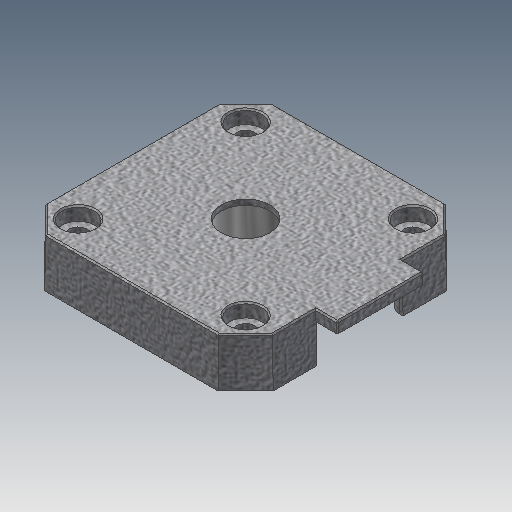
# Autodesk Inventor part: Nema 17 Base Cap
Saved by Autodesk Inventor 2020.2 (Build 242310000, 310)
## iProperties
Created: 2020-01-17
Part Number: Nema 17 Base Cap
Material: Aluminum 6061
Document SubType Name: Modeling
Designer: james
Density: 2.7 g/cm^3
Appearance: Aluminum Cast
Mass: 22.7 g
Surface Area: 71.1651 cm^2
Volume: 8.4074 cm^3
Author: james
Autodesk Inventor part; units mm, degrees
ref_plane "YZ Plane" through (0, 0, 0) normal (1, 0, 0) x (0, 1, 0)
ref_plane "XZ Plane" through (0, 0, 0) normal (0, 1, 0) x (-1, 0, 0)
ref_plane "XY Plane" through (0, 0, 0) normal (0, 0, 1) x (1, 0, 0)
sketch "Sketch11" plane through (0, 0, 0) normal (0, 1, 0) x (-1, 0, 0)
  line L0 (-16, 21) -> (16, 21)
  line L1 (21, 16) -> (21, -16)
  line L2 (16, -21) -> (-16, -21)
  line L3 (-21, -16) -> (-21, 16)
  line L4 (-21, 21) -> (21, -21) construction
  line L5 (21, 21) -> (-21, -21) construction
  line L6 (21, -16) -> (16, -21)
  line L7 (-16, -21) -> (-21, -16)
  line L8 (-21, 16) -> (-16, 21)
  line L9 (16, 21) -> (21, 16)
  point P0 (0, 0)
  dimension "d82" = 42
  dimension "d83" = 5
  dimension "d84" = 5
  dimension "d85" = 5
  dimension "d86" = 5
  dimension "d87" = 5
  dimension "d88" = 5
  dimension "d89" = 5
  dimension "d90" = 5
  constraints: 20 end point, 8 point on line, 2 midpoint, 2 parallel, 2 perpendicular, 1 horizontal
  measures "d82" distance between parallel lines of L0 L2
  measures "d83" distance of L1.end L4.end
  measures "d84" distance of L2.start L4.end
  measures "d85" distance of L2.end L5.end
  measures "d86" distance of L3.start L5.end
  measures "d87" distance of L3.end L4.start
  measures "d88" distance of L0.start L4.start
  measures "d89" distance of L0.end L5.start
  measures "d90" distance of L1.start L5.start
extrude "Extrusion7" add sketch "Sketch11" against normal blind 9 draft 1
sketch "Sketch13" plane through (0, -9, 0) normal (0, -1, 0) x (1, 0, 0)
  circle A0 centre (0, 0) radius 13
  line L0 (-8.0772, 19.5) -> (8.0772, 19.5)
  line L1 (8.0772, 19.5) -> (19.5, 8.0772)
  line L2 (19.5, 8.0772) -> (19.5, -8.0772)
  line L3 (19.5, -8.0772) -> (8.0772, -19.5)
  line L4 (8.0772, -19.5) -> (-8.0772, -19.5)
  line L5 (-8.0772, -19.5) -> (-19.5, -8.0772)
  line L6 (-19.5, -8.0772) -> (-19.5, 8.0772)
  line L7 (-19.5, 8.0772) -> (-8.0772, 19.5)
  dimension "d96" = 26
  dimension "d97" = 39
  constraints: 16 end point, 2 coincident, 1 centre point, 1 vertical, 17 other
  measures "d96" diameter of A0
  measures "d97" distance between parallel lines of L2 L6
extrude "Extrusion9" cut sketch "Sketch13" against normal blind 7
sketch "Sketch14" plane through (0, -9, 0) normal (0, -1, 0) x (1, 0, 0)
  circle A0 centre (0, 0) radius 13 projected
extrude "Extrusion10" add sketch "Sketch14" along normal blind 1
sketch "Sketch15" plane through (0, -10, 0) normal (0, -1, 0) x (1, 0, 0)
  circle A0 centre (0, 0) radius 8
  dimension "d102" = 16
  constraints: 1 centre point, 1 coincident
  measures "d102" diameter of A0
extrude "Extrusion11" cut sketch "Sketch15" against normal blind 8.25
sketch "Sketch17" plane through (0, -1.75, 0) normal (0, -1, 0) x (1, 0, 0)
  circle A0 centre (0, 0) radius 6
  dimension "d112" = 12
  constraints: 1 centre point, 1 coincident
  measures "d112" diameter of A0
extrude "Extrusion12" cut sketch "Sketch17" against normal blind 0.75
sketch "Sketch18" plane through (0, 0, 0) normal (0, 1, 0) x (1, 0, 0)
  line L0 (-15.5, 15.5) -> (15.5, 15.5) construction
  line L1 (15.5, 15.5) -> (15.5, -15.5) construction
  line L2 (15.5, -15.5) -> (-15.5, -15.5) construction
  line L3 (-15.5, -15.5) -> (-15.5, 15.5) construction
  line L4 (-15.5, 15.5) -> (15.5, -15.5) construction
  line L5 (15.5, 15.5) -> (-15.5, -15.5) construction
  point P0 (0, 0)
  point P1 (0, 0)
  dimension "d115" = 31
  dimension "d124" = 31
  constraints: 12 end point, 2 midpoint, 1 coincident, 1 horizontal, 1 vertical
  measures "d115" distance of L0.start L0.end
  measures "d124" distance of L2.end L0.start
hole "Hole6" at (-15.5, 0, -15.5) at (15.5, 0, -15.5) at (15.5, 0, 15.5) at (-15.5, 0, 15.5) direction (0, -1, 0) diameter 3.4 end through all counterbore diameter 6 counterbore depth 2.5 clearance for "Socket Head Cap Screw" size "M3" standard "Ansi Metric M Profile"
chamfer "Chamfer1" distance 0.25 distance2 1 1 edges at (-8, -10, 0) measured on face at (11.1299, -10, -1.6752)
chamfer "Chamfer2" distance 0.25 angle 45 9 edges at (-13, -10, 0) (-21, 0, 0) (-18.5, 0, 18.5) (0, 0, 21) (18.5, 0, 18.5) (21, 0, 0) (18.5, 0, -18.5) (0, 0, -21) (-18.5, 0, -18.5)
sketch "Sketch19" plane through (0, 0, 0) normal (0, 1, 0) x (1, 0, 0)
  point P0 (0, 0)
  point P1 (0, 0)
  constraints: 1 coincident
hole "Hole7" at (0, 0, 0) direction (0, -1, 0) diameter 9 end through all
sketch "Sketch20" plane through (0, -2, 0) normal (0, -1, 0) x (1, 0, 0)
  line L0 (-8.0772, -19.5) -> (-12.5352, -15.042) projected
  line L1 (-15.042, -12.5352) -> (-19.5, -8.0772) projected
  arc A0 (-12.0208, -15.5563) -> (-15.5563, -12.0208) centre (-15.5, -15.5) ccw
  circle A1 centre (-15.5, -15.5) radius 1.7 projected
  line L2 (-12.5352, -15.042) -> (-15.042, -12.5352) projected
  point P0 (0, 0)
  dimension "d138" = 5
  constraints: 2 point on circle, 2 point on line, 1 centre point, 1 concentric
  measures "d138" distance of A0.end A0.start
extrude "Extrusion13" add sketch "Sketch20" along normal blind 1 contours L0 L2 L1 A0
sketch "Sketch21" plane through (0, -2, 0) normal (0, 1, 0) x (1, 0, 0)
  arc A0 (-15.042, 12.5352) -> (-12.5352, 15.042) centre (-15.5, 15.5) ccw projected
  line L0 (-15.042, 12.5352) -> (-12.5352, 15.042) projected
  point P0 (0, 0)
extrude "Extrusion14" cut sketch "Sketch21" against normal up to surface (0.5 mm away)
pattern_circular "Circular Pattern1" count 4 over 360 about axis through (0, -10, 0) along (0, 1, 0) of "Extrusion14", "Extrusion13"
sketch "Sketch22" plane through (0, 0, 0) normal (0, 1, 0) x (1, 0, 0)
  line L0 (21, 8) -> (25, 8)
  line L1 (25, 8) -> (25, -8)
  line L2 (25, -8) -> (21, -8)
  line L3 (21, -8) -> (21, 8)
  point P0 (0, 0)
  point P1 (21, 0)
  dimension "d146" = 4
  dimension "d147" = 16
  dimension "d148" = 21
  constraints: 8 end point, 2 parallel, 1 horizontal, 1 horizontal alignment, 1 midpoint, 1 perpendicular
  measures "d146" distance of L0.start L0.end
  measures "d147" distance of L0.end L1.end
  measures "d148" distance from line of L3 point (0, 0)
extrude "Extrusion15" add sketch "Sketch22" against normal blind 3
sketch "Sketch23" plane through (21, 0, -8) normal (-1, 0, 0) x (0, 0, 1)
  line L0 (16, -0.2457) -> (0, -0.2457) projected
  line L1 (16, 0) -> (16, -0.2457) projected
  line L2 (0, 0) -> (16, 0) projected
  line L3 (0, 0) -> (0, -0.2457) projected
  point P0 (8, 0)
extrude "Extrusion16" add sketch "Sketch23" along normal up to next
sketch "Sketch24" plane through (0, -9, 0) normal (0, -1, 0) x (1, 0, 0)
  line L0 (25, -8) -> (25, 8) projected
  line L1 (25, -8) -> (19.5, -8)
  line L2 (19.5, -8) -> (19.5, 8)
  line L3 (19.5, 8) -> (25, 8)
  line L4 (25, 8) -> (25, -8)
  line L5 (25, 8) -> (21.0524, 8) projected
  line L6 (19.5, 8.0772) -> (19.5, -8.0772) projected
  point P0 (0, 0)
  constraints: 8 end point, 2 collinear, 2 parallel, 1 horizontal, 1 perpendicular
extrude "Extrusion17" cut sketch "Sketch24" against normal up to surface (7 mm away)
sketch "Sketch25" plane through (0, -2, 0) normal (0, -1, 0) x (1, 0, 0)
  line L0 (17, -7) -> (24, -7)
  line L1 (24, -7) -> (24, 7)
  line L2 (24, 7) -> (17, 7)
  line L3 (17, 7) -> (17, -7)
  line L4 (25, 8) -> (25, -8) projected
  point P0 (0, 0)
  point P1 (24, 0)
  point P2 (25, 0)
  dimension "d155" = 7
  dimension "d156" = 14
  dimension "d157" = 1
  constraints: 8 end point, 2 midpoint, 2 parallel, 1 horizontal, 1 horizontal alignment, 1 perpendicular
  measures "d155" distance of L2.end L1.end
  measures "d156" distance of L1.end L0.end
  measures "d157" distance between parallel lines of L4 L1
extrude "Extrusion18" cut sketch "Sketch25" against normal blind 1.8
fillet "Fillet8" radius 0.5 4 edges at (17, -1.1, -7) (24, -1.1, -7) (24, -1.1, 7) (17, -1.1, 7)
chamfer "Chamfer3" distance 0.25 angle 45 5 edges at (22.875, 0, 8) (25, 0, 0) (22.875, 0, -8) (25, -1, -8) (25, -1, 8)
fillet "Fillet9" radius 2 2 edges at (19.5, -5.5, 8) (19.5, -5.5, -8)
fillet "Fillet10" radius 2 2 edges at (19.5, -5.5, 8.0772) (19.5, -5.5, -8.0772)
chamfer "Chamfer4" distance 0.25 angle 45 4 edges at (-15.5, 0, -18.5) (15.5, 0, -18.5) (15.5, 0, 12.5) (-15.5, 0, 12.5)
equation "\"d84\" = d83"
equation "\"d85\" = d83"
equation "\"d86\" = d85"
equation "\"d87\" = d83"
equation "\"d88\" = d87"
equation "\"d89\" = d83"
equation "\"d90\" = d89"
body "Solid6"
